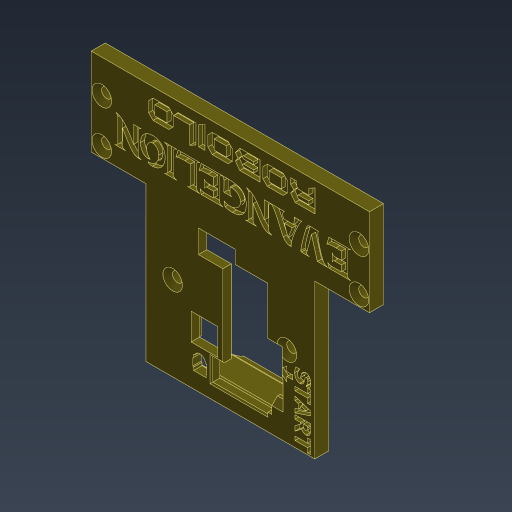
# Autodesk Inventor part: ceil
Saved by Autodesk Inventor 2023 (Build 270158000, 158)
## iProperties
Created: 2025-04-29
Part Number: ceil
Material: Generic
Document SubType Name: Modeling
Designer: szymo
Density: 1 g/cm^3
Appearance: Default(3)
Mass: 14.6413 g
Surface Area: 135.463 cm^2
Volume: 14.6413 cm^3
Author: szymo
Autodesk Inventor part; units mm, degrees
ref_plane "YZ Plane" through (0, 0, 0) normal (1, 0, 0) x (0, 1, 0)
ref_plane "XZ Plane" through (0, 0, 0) normal (0, 1, 0) x (-1, 0, 0)
ref_plane "XY Plane" through (0, 0, 0) normal (0, 0, 1) x (1, 0, 0)
ref_plane "Work Plane1" through (0, 0, 0) normal (0, 0, 1) x (1, 0, 0)
sketch "Sketch1" plane through (0, 0, 0) normal (0, 0, 1) x (1, 0, 0)
  spline S0 degree 2 poles (-9.1441, -18.5243) (-10.521, -19.0902) (-11.8979, -18.5243) knots 0 0 0 1 1 1 weights 1 1.096933 1
  line L0 (-16.1375, -18.5243) -> (-11.8979, -18.5243)
  line L1 (-16.1375, -20.5243) -> (-16.1375, -18.5243)
  line L2 (16.1375, -20.5243) -> (-16.1375, -20.5243)
  line L3 (16.1375, 6.7419) -> (16.1375, -20.5243)
  line L4 (16.1375, 6.7419) -> (16.1375, 10.5894)
  line L5 (8.6375, -18.5243) -> (8.6375, 6.7419)
  line L6 (-9.1441, -18.5243) -> (8.6375, -18.5243)
  circle A0 centre (12.3875, -16.7743) radius 2.75
  circle A1 centre (12.3875, -1.2581) radius 2.75
  line L7 (-53.5375, -20.5243) -> (-53.5375, -18.5243)
  line L8 (-53.5375, -18.5243) -> (-54.5271, -18.5243)
  line L9 (-54.5271, -18.5243) -> (-57.2809, -18.5243)
  line L10 (-57.2809, -18.5243) -> (-75.3625, -18.5243)
  line L11 (-75.3625, -18.5243) -> (-75.3625, 6.7419)
  line L12 (-82.8625, 6.7419) -> (-75.3625, 6.7419)
  line L13 (-82.8625, 6.7419) -> (-82.8625, -20.5243)
  line L14 (-82.8625, -20.5243) -> (-53.5375, -20.5243)
  circle A2 centre (-79.1125, -16.7743) radius 2.75
  circle A3 centre (-79.1125, -1.2581) radius 2.75
  arc A4 (-51.8547, -63.7607) -> (-50.5875, -61.8998) centre (-52.5875, -61.8998) ccw
  line L15 (-50.5875, -61.8998) -> (-50.5875, -36.1001)
  line L16 (-50.5875, -36.1001) -> (-56.7375, -36.1001)
  line L17 (-56.7375, -36.1001) -> (-56.7375, -20.5243)
  line L18 (-56.7375, -20.5243) -> (-61.3875, -20.5243)
  line L19 (-61.3875, -75.3243) -> (-61.3875, -20.5243)
  line L20 (-47.5875, -75.3243) -> (-61.3875, -75.3243)
  line L21 (-47.5875, -70.3243) -> (-47.5875, -75.3243)
  line L22 (-47.5875, -70.3243) -> (-50.6091, -70.3243)
  arc A5 (-51.8547, -63.7607) -> (-50.6091, -70.3243) centre (-50.6091, -66.9243) ccw
  circle A6 centre (-53.8875, -45.365) radius 2.75
  circle A7 centre (-13.2119, -46.6658) radius 2.75
  arc A8 (-14.1375, -70.3243) -> (-16.1375, -72.3243) centre (-14.1375, -72.3243) ccw
  line L23 (-16.1375, -72.3243) -> (-16.1375, -75.3243)
  line L24 (-16.1375, -75.3243) -> (-5.3375, -75.3243)
  line L25 (-5.3375, -20.5243) -> (-5.3375, -75.3243)
  line L26 (-16.1375, -20.5243) -> (-5.3375, -20.5243)
  line L27 (-16.1375, -58.1001) -> (-16.1375, -20.5243)
  line L28 (-16.1375, -58.1001) -> (-9.9875, -58.1001)
  line L29 (-9.9875, -58.1001) -> (-9.9875, -63.9243)
  arc A9 (-9.9875, -63.9243) -> (-10.3793, -65.8628) centre (-8.4794, -65.238) ccw
  arc A10 (-10.2091, -66.9243) -> (-10.3793, -65.8628) centre (-13.6102, -66.9254) ccw
  arc A11 (-13.6102, -70.3243) -> (-10.2091, -66.9243) centre (-13.6102, -66.9232) ccw
  line L30 (-13.6102, -70.3243) -> (-14.1375, -70.3243)
  line L31 (-5.3375, -75.3243) -> (-61.3875, -75.3243)
  line L32 (16.1375, 10.5894) -> (-82.3497, 10.5894)
  line L33 (-5.3375, -20.5243) -> (-5.3375, -75.3243)
  line L34 (-5.3375, -75.3243) -> (-3.3375, -75.3243)
  line L35 (-3.3375, -20.5243) -> (-3.3375, -75.3243)
  line L36 (-5.3375, -20.5243) -> (-3.3375, -20.5243)
  line L37 (-61.3875, -75.3243) -> (-61.3875, -20.5243)
  line L38 (-61.3875, -20.5243) -> (-63.3875, -20.5243)
  line L39 (-63.3875, -75.3243) -> (-63.3875, -73.1158)
  line L40 (-61.3875, -75.3243) -> (-63.3875, -75.3243)
  spline S1 degree 2 poles (-63.3875, -70.8783) (-63.0299, -71.9971) (-63.3875, -73.1158) knots 0 0 0 1 1 1 weights 1 1.055366 1
  line L41 (-63.3875, -70.8783) -> (-63.3875, -20.5243)
  line L42 (-63.3875, -73.1158) -> (-63.3875, -70.8783)
  line L43 (-22.0095, -69.5462) -> (-22.0095, -31.5462)
  line L44 (-34.0095, -69.5462) -> (-22.0095, -69.5462)
  line L45 (-34.0095, -31.5462) -> (-34.0095, -69.5462)
  line L46 (-22.0095, -31.5462) -> (-34.0095, -31.5462)
  line L47 (-41.7145, -65.6143) -> (-41.7145, -68.3743)
  line L48 (-41.7145, -68.3743) -> (-41.9645, -68.6243)
  line L49 (-41.9645, -68.6243) -> (-41.9645, -69.6243)
  line L50 (-41.9645, -69.6243) -> (-46.4645, -69.6243)
  line L51 (-46.4645, -69.6243) -> (-46.4645, -68.6243)
  line L52 (-46.4645, -68.6243) -> (-46.4645, -68.6243)
  line L53 (-46.7145, -68.3743) -> (-46.7145, -65.8743)
  line L54 (-46.7145, -65.8743) -> (-46.4645, -65.6243)
  line L55 (-46.4645, -65.6243) -> (-46.4645, -64.6243)
  line L56 (-46.4645, -68.6243) -> (-46.4645, -68.6243)
  line L57 (-46.4645, -68.6243) -> (-46.7145, -68.3743)
  line L58 (-42.7044, -64.6243) -> (-41.7145, -65.6143)
  line L59 (-46.4645, -64.6243) -> (-42.7044, -64.6243)
  line L60 (-36.1845, -69.2743) -> (-36.1845, -63.2743)
  line L61 (-36.1845, -69.2743) -> (-37.8845, -69.2743)
  line L62 (-39.0845, -68.4743) -> (-39.0845, -64.0743)
  line L63 (-36.1845, -63.2743) -> (-37.8845, -63.2743)
  line L64 (-37.8845, -63.2743) -> (-37.8845, -63.7743)
  line L65 (-38.7345, -63.7743) -> (-37.8845, -63.7743)
  line L66 (-38.7345, -63.7743) -> (-38.9845, -64.0243)
  line L67 (-37.8845, -69.2743) -> (-37.8845, -68.7743)
  line L68 (-38.9845, -68.5243) -> (-38.7345, -68.7743)
  line L69 (-38.7345, -68.7743) -> (-37.8845, -68.7743)
  line L70 (-38.9845, -68.5243) -> (-38.7345, -68.7743)
  line L71 (-38.9845, -68.4743) -> (-39.0845, -68.4743)
  line L72 (-38.9845, -68.4743) -> (-38.9845, -68.5243)
  line L73 (-38.9845, -64.0743) -> (-39.0845, -64.0743)
  line L74 (-38.9845, -64.0243) -> (-38.9845, -64.0743)
  line L75 (-38.8144, -60.2785) -> (-38.8144, -52.7785)
  line L76 (-46.3195, -60.2785) -> (-38.8144, -60.2785)
  line L77 (-46.3195, -52.7785) -> (-46.3195, -60.2785)
  line L78 (-38.8144, -52.7785) -> (-46.3195, -52.7785)
  line L79 (-32.6145, -25.8443) -> (-43.7145, -25.8443)
  line L80 (-43.7145, -25.8443) -> (-43.7145, -28.0943)
  line L81 (-43.7145, -28.0943) -> (-43.7145, -29.7943)
  line L82 (-43.7145, -25.8443) -> (-43.7145, -32.0443)
  line L83 (-43.7145, -32.0443) -> (-42.7145, -32.0443)
  line L84 (-42.7145, -32.0443) -> (-32.6145, -32.0443)
  line L85 (-42.7145, -32.0443) -> (-32.6145, -32.0443)
  line L86 (-32.6145, -25.8443) -> (-32.6145, -32.0443)
  line L87 (-17.8595, -56.3243) -> (-17.8595, -49.5243)
  line L88 (-20.8595, -56.3243) -> (-17.8595, -56.3243)
  line L89 (-20.8595, -49.5243) -> (-20.8595, -56.3243)
  line L90 (-17.8595, -49.5243) -> (-20.8595, -49.5243)
  line L91 (-17.6095, -63.5243) -> (-17.6095, -57.5243)
  line L92 (-17.6095, -63.5243) -> (-19.3095, -63.5243)
  line L93 (-19.3095, -63.5243) -> (-19.3095, -63.0243)
  line L94 (-20.1595, -63.0243) -> (-19.3095, -63.0243)
  line L95 (-20.4095, -62.7743) -> (-20.1595, -63.0243)
  line L96 (-20.4095, -62.7243) -> (-20.4095, -62.7743)
  line L97 (-20.4095, -62.7243) -> (-20.5095, -62.7243)
  line L98 (-20.4095, -62.7243) -> (-20.5095, -62.7243)
  line L99 (-20.5095, -62.7243) -> (-20.5095, -58.3243)
  line L100 (-17.6095, -57.5243) -> (-19.3095, -57.5243)
  line L101 (-19.3095, -57.5243) -> (-19.3095, -58.0243)
  line L102 (-20.1595, -58.0243) -> (-19.3095, -58.0243)
  line L103 (-20.1595, -58.0243) -> (-20.4095, -58.2743)
  line L104 (-20.4095, -58.2743) -> (-20.4095, -58.3243)
  line L105 (-20.4095, -58.3243) -> (-20.5095, -58.3243)
  line L106 (-19.6095, -66.9243) -> (-19.6095, -66.6743)
  line L107 (-19.6095, -66.3743) -> (-19.6095, -66.1243)
  line L108 (-19.9095, -66.1243) -> (-20.9095, -66.1243)
  line L109 (-21.2095, -66.3743) -> (-21.2095, -66.1243)
  line L110 (-21.2095, -66.9243) -> (-21.2095, -66.6743)
  line L111 (-19.9095, -66.9243) -> (-20.9095, -66.9243)
  line L112 (-19.9095, -67.4743) -> (-20.9095, -67.4743)
  line L113 (-19.9095, -68.2743) -> (-20.9095, -68.2743)
  line L114 (-19.6095, -68.2743) -> (-19.6095, -68.0243)
  line L115 (-19.6095, -67.7243) -> (-19.6095, -67.4743)
  line L116 (-21.2095, -67.7243) -> (-21.2095, -67.4743)
  line L117 (-21.2095, -68.2743) -> (-21.2095, -68.0243)
  line L118 (-19.6095, -65.6243) -> (-19.6095, -65.3743)
  line L119 (-19.6095, -65.0743) -> (-19.6095, -64.8243)
  line L120 (-19.9095, -64.8243) -> (-20.9095, -64.8243)
  line L121 (-19.9095, -65.6243) -> (-20.9095, -65.6243)
  line L122 (-21.2095, -65.6243) -> (-21.2095, -65.3743)
  line L123 (-21.2095, -65.0743) -> (-21.2095, -64.8243)
  line L124 (-20.0095, -70.2743) -> (-20.0095, -29.5462)
  line L125 (-20.0095, -29.5462) -> (-36.0095, -29.5462)
  line L126 (-36.0095, -29.5462) -> (-36.0095, -70.2743)
  line L127 (-31.6145, -24.8443) -> (-44.7145, -24.8443)
  line L128 (-44.7145, -24.8443) -> (-44.7145, -33.0443)
  line L129 (-44.7145, -33.0443) -> (-31.6145, -33.0443)
  line L130 (-31.6145, -33.0443) -> (-31.6145, -24.8443)
  line L131 (-21.8595, -48.5243) -> (-21.8595, -57.3243)
  line L132 (-21.8595, -57.3243) -> (-16.8595, -57.3243)
  line L133 (-16.8595, -57.3243) -> (-16.8595, -48.5243)
  line L134 (-16.8595, -48.5243) -> (-21.8595, -48.5243)
  line L135 (-16.6095, -64.5243) -> (-21.5095, -64.5243)
  line L136 (-21.5095, -64.5243) -> (-21.5095, -56.5243)
  line L137 (-21.5095, -56.5243) -> (-16.6095, -56.5243)
  line L138 (-16.6095, -56.5243) -> (-16.6095, -64.5243)
  line L139 (-40.0845, -70.2743) -> (-35.1845, -70.2743)
  line L140 (-35.1845, -70.2743) -> (-35.1845, -62.2743)
  line L141 (-35.1845, -62.2743) -> (-40.0845, -62.2743)
  line L142 (-40.0845, -62.2743) -> (-40.0845, -70.2743)
  line L143 (-37.8144, -61.2785) -> (-37.8144, -51.7785)
  line L144 (-37.8144, -51.7785) -> (-47.3195, -51.7785)
  line L145 (-47.3195, -51.7785) -> (-47.3195, -61.2785)
  line L146 (-47.3195, -61.2785) -> (-37.8144, -61.2785)
  circle A12 centre (-44.2145, -65.3243) radius 0.4
  circle A13 centre (-44.2145, -65.3243) radius 2
  line L147 (-18.6095, -69.2743) -> (-22.2095, -69.2743)
  line L148 (-22.2095, -69.2743) -> (-22.2095, -64.5243)
  line L149 (-22.2095, -64.5243) -> (-18.6095, -64.5243)
  line L150 (-18.6095, -64.5243) -> (-18.6095, -69.2743)
  line L151 (-82.8625, 10.5894) -> (-75.3625, 10.5894)
  line L152 (-82.8625, 6.7419) -> (-82.8625, 10.5894)
  line L153 (-20.0095, -70.2743) -> (-36.0095, -70.2743)
  line L154 (-36.0095, -70.2743) -> (-41.4052, -70.2743) construction
  point P0 (0, 0)
  point P1 (-37.6345, -70.2743)
  point P2 (-36.0095, -70.2743)
  point P3 (-36.0095, -62.2743)
  point P4 (-36.0095, -33.0443)
  point P5 (-31.6145, -29.5462)
  point P6 (-20.0095, -48.5243)
  point P7 (-16.6095, -58.3243)
  point P8 (-20.0095, -69.2743)
  point P9 (-42.8879, -64.6243)
  point P10 (-46.088, -64.6243)
  point P11 (-20.0095, -64.5243)
  point P12 (-16.8595, -56.5243)
  point P13 (-20.0095, -56.5243)
  point P14 (-20.0095, -57.3243)
  point P15 (-21.5095, -57.3243)
  point P16 (-42.2269, -65.1019)
  dimension "d97" = 1
  dimension "d98" = 1
  dimension "d99" = 1
  dimension "d100" = 1
  dimension "d101" = 1
  dimension "d102" = 1
  dimension "d103" = 4
  dimension "d104" = 1
  dimension "d105" = 1
  dimension "d106" = 1
  dimension "d107" = 1
  dimension "d108" = 1
  dimension "d109" = 1
  dimension "d110" = 1
  dimension "d111" = 1
  dimension "d112" = 1
  dimension "d113" = 1
  dimension "d114" = 1
  dimension "d153" = 2
  dimension "d154" = 0.7281
  dimension "d155" = 0
  constraints: 234 end point, 15 vertical, 12 horizontal, 11 parallel, 6 perpendicular, 3 collinear, 2 centre point, 1 coincident, 1 midpoint, 1 point on line, 165 other
  measures "d97" distance between parallel lines of L127 L79
  measures "d98" distance between parallel lines of L128 L80
  measures "d99" distance between parallel lines of L129 L84
  measures "d100" distance between parallel lines of L130 L86
  measures "d101" distance between parallel lines of L90 L134
  measures "d102" distance between parallel lines of L76 L146
  measures "d103" diameter of A13
  measures "d104" distance between parallel lines of L138 L91
  measures "d105" distance between parallel lines of L135 L92
  measures "d106" distance between parallel lines of L136 L99
  measures "d107" distance between parallel lines of L100 L137
  measures "d108" distance from line of L61 point (-37.635, -70.274)
  measures "d109" distance between parallel lines of L142 L62
  measures "d110" distance between parallel lines of L63 L141
  measures "d111" distance between parallel lines of L140 L60
  measures "d112" distance between parallel lines of L150 L114
  measures "d113" distance between parallel lines of L147 L113
  measures "d114" distance from line of L148 L117.end
  measures "d153" distance between parallel lines of L45 L126
  measures "d154" distance between parallel lines of L153 L44
  measures "d155" distance between parallel lines of L154 L139
extrude "Extrusion1" add sketch "Sketch1" along normal blind 5 contours L2 L27 L28 L29 A9 A10 A11 L30 A8 L23 L31 L21 L22 A5 A4 L15 L16 L17 L14 L7 L8 L9 L10 L11 L12 L152 L151 L32 L4 L3 | L35 L34 L25 L2 | L25 L24 L23 A8 L30 A11 A10 A9 L29 L28 L27 L2 | L20 L19 L14 L17 L16 L15 A4 A5 L22 L21 | L40 L39 S1 L41 L14 L19 | L12 L11 L10 L9 L8 L7 L14 L13 | L42 S1 | A0 | A1 | A2 | A3 | A6 | A7
sketch "Sketch6" plane through (0, 0, 0) normal (0, 0, -1) x (-1, 0, 0)
  circle A0 centre (50.6091, -66.9243) radius 2
  arc A1 (16.1375, -65.8429) -> (16.1375, -68.0058) centre (13.6091, -66.9243) ccw
  circle A2 centre (50.6091, -66.9243) radius 4
  circle A3 centre (13.6091, -66.9243) radius 3.5
  point P0 (0, 0)
  dimension "d83" = 8
  dimension "d84" = 7
  constraints: 4 centre point, 2 coincident, 2 point on circle, 6 other
  measures "d83" diameter of A2
  measures "d84" diameter of A3
extrude "Extrusion5" cut sketch "Sketch6" against normal blind 2 contours A0 | A2 | A3
ref_plane "Work Plane2" through (-16.6375, -70.0451, -5.2063) normal (-1, 0, 0) x (0, -0.9586871, -0.2844628)
sketch "Sketch7" plane through (-16.6375, -70.0451, -5.2063) normal (-1, 0, 0) x (0, -0.9586871, -0.2844628)
  line L0 (3.5801, 6.493) -> (7.0645, -5.2498)
  arc A0 (6.3902, -6.493) -> (-6.4635, -1.1345) centre (-4.8206, -15.2895) ccw
  line L1 (-0.6539, 3.1854) -> (-1.2133, 5.0707)
  line L2 (7.3489, -6.2085) -> (6.3902, -6.493)
  line L3 (1.4628, 5.8648) -> (3.5801, 6.493)
  line L4 (-0.6822, 5.2283) -> (1.4628, 5.8648)
  line L5 (-0.6822, 5.2283) -> (-1.2133, 5.0707)
  line L6 (-0.1588, 5.3836) -> (2.3155, -2.9551)
  line L7 (7.0645, -5.2498) -> (7.3489, -6.2085)
  line L8 (-0.1588, 5.3836) -> (-1.2133, 5.0707)
  point P0 (-68.6323, -14.934)
  dimension "d88" = 1
  dimension "d89" = 1.1
  dimension "d150" = 3.9
  constraints: 18 end point, 4 point on circle, 2 perpendicular, 2 point on line, 1 centre point, 1 collinear, 14 other
  measures "d88" distance of L2.start L2.end
  measures "d89" distance between parallel lines of L1 L6
  measures "d150" distance between parallel lines of L6 L0
extrude "Extrusion6" add sketch "Sketch7" along normal blind 30.45
chamfer "Chamfer8" distance 2 angle 45 4 edges at (-18.4345, -48.5243, 5) (-16.8595, -52.5243, 5) (-16.6095, -60.5243, 5) (-17.6095, -64.5243, 5)
chamfer "Chamfer9" distance 0.5 angle 45 3 edges at (-30.047, -70.2743, 5) (-40.0845, -66.2743, 5) (-38.047, -62.2743, 5)
sketch "Sketch5" plane through (0, 0, 5) normal (0, 0, 1) x (1, 0, 0)
  spline S0 degree 2 poles (-9.1441, -18.5243) (-10.521, -19.0902) (-11.8979, -18.5243) knots 0 0 0 1 1 1 weights 1 1.096933 1
  line L0 (-16.1375, -18.5243) -> (-11.8979, -18.5243)
  line L1 (-16.1375, -20.5243) -> (-16.1375, -18.5243)
  line L2 (16.1375, -20.5243) -> (-16.1375, -20.5243)
  line L3 (16.1375, 6.7419) -> (16.1375, -20.5243)
  line L4 (16.1375, 6.7419) -> (8.6375, 6.7419)
  line L5 (8.6375, -18.5243) -> (8.6375, 6.7419)
  line L6 (-9.1441, -18.5243) -> (8.6375, -18.5243)
  circle A0 centre (12.3875, -16.7743) radius 2.75
  circle A1 centre (12.3875, -1.2581) radius 2.75
  line L7 (-53.5375, -20.5243) -> (-53.5375, -18.5243)
  line L8 (-53.5375, -18.5243) -> (-54.5271, -18.5243)
  line L9 (-54.5271, -18.5243) -> (-57.2809, -18.5243)
  line L10 (-57.2809, -18.5243) -> (-75.3625, -18.5243)
  line L11 (-75.3625, -18.5243) -> (-75.3625, 6.7419)
  line L12 (-82.8625, 6.7419) -> (-75.3625, 6.7419)
  line L13 (-82.8625, 6.7419) -> (-82.8625, -20.5243)
  line L14 (-82.8625, -20.5243) -> (-53.5375, -20.5243)
  circle A2 centre (-79.1125, -16.7743) radius 2.75
  circle A3 centre (-79.1125, -1.2581) radius 2.75
  arc A4 (-51.8547, -63.7607) -> (-50.5875, -61.8998) centre (-52.5875, -61.8998) ccw
  line L15 (-50.5875, -61.8998) -> (-50.5875, -36.1001)
  line L16 (-50.5875, -36.1001) -> (-56.7375, -36.1001)
  line L17 (-56.7375, -36.1001) -> (-56.7375, -20.5243)
  line L18 (-56.7375, -20.5243) -> (-61.3875, -20.5243)
  line L19 (-61.3875, -75.3243) -> (-61.3875, -20.5243)
  line L20 (-47.5875, -75.3243) -> (-61.3875, -75.3243)
  line L21 (-47.5875, -70.3243) -> (-47.5875, -75.3243)
  line L22 (-47.5875, -70.3243) -> (-50.6091, -70.3243)
  arc A5 (-51.8547, -63.7607) -> (-50.6091, -70.3243) centre (-50.6091, -66.9243) ccw
  circle A6 centre (-53.8875, -45.365) radius 2.75
  circle A7 centre (-13.2119, -46.6658) radius 2.75
  arc A8 (-14.1375, -70.3243) -> (-16.1375, -72.3243) centre (-14.1375, -72.3243) ccw
  line L23 (-16.1375, -72.3243) -> (-16.1375, -75.3243)
  line L24 (-16.1375, -75.3243) -> (-5.3375, -75.3243)
  line L25 (-5.3375, -20.5243) -> (-5.3375, -75.3243)
  line L26 (-16.1375, -20.5243) -> (-5.3375, -20.5243)
  line L27 (-16.1375, -58.1001) -> (-16.1375, -20.5243)
  line L28 (-16.1375, -58.1001) -> (-9.9875, -58.1001)
  line L29 (-9.9875, -58.1001) -> (-9.9875, -63.9243)
  arc A9 (-9.9875, -63.9243) -> (-10.3793, -65.8628) centre (-8.4794, -65.238) ccw
  arc A10 (-10.2091, -66.9243) -> (-10.3793, -65.8628) centre (-13.6102, -66.9254) ccw
  arc A11 (-13.6102, -70.3243) -> (-10.2091, -66.9243) centre (-13.6102, -66.9232) ccw
  line L30 (-13.6102, -70.3243) -> (-14.1375, -70.3243)
  point P0 (0, 0)
  point P1 (12.3875, -1.2581)
  point P2 (12.3875, -16.7743)
  dimension "d108" = 1
  constraints: 8 coincident
hole "Hole1" at (-53.8875, -45.365, 5) at (-13.2119, -46.6658, 5) at (12.3875, -1.2581, 5) at (12.3875, -16.7743, 5) at (-79.1125, -16.7743, 5) at (-79.1125, -1.2581, 5) direction (0, 0, -1) diameter 3.6 depth 8.8 countersink diameter 7 countersink angle 90 clearance for "Countersunk Flat Head Screw ISO 2009/7046" size "M3" standard "ISO"
fillet "Fillet1" radius 0.6 8 edges at (-47.0875, -71.4243, -4.349) (-47.0875, -73.0917, -10.8349) (-47.0875, -74.8243, -13.2489) (-16.6375, -73.0917, -10.8349) (-16.6375, -71.4243, -4.349) (-16.6375, -74.8243, -13.2489) (-31.8625, -74.3243, -13.2489) (-31.8625, -71.4243, -8.698)
sketch "Sketch8" plane through (0, 0, 0) normal (0, 0, -1) x (-1, 0, 0)
  line L0 (50.6091, -69.9243) -> (13.6091, -69.9243)
  arc A0 (50.6091, -69.9243) -> (50.6091, -63.9243) centre (50.6091, -66.9243) ccw
  line L1 (49.1091, -63.9243) -> (50.6091, -63.9243)
  arc A1 (47.1091, -61.9243) -> (49.1091, -63.9243) centre (49.1098, -61.9236) ccw
  line L2 (47.1091, -17.9243) -> (47.1091, -61.9243)
  line L3 (17.1091, -17.9243) -> (47.1091, -17.9243)
  line L4 (17.1091, -61.9243) -> (17.1091, -17.9243)
  arc A2 (15.1091, -63.9243) -> (17.1091, -61.9243) centre (15.1083, -61.9236) ccw
  line L5 (13.6091, -63.9243) -> (15.1091, -63.9243)
  arc A3 (13.6091, -63.9243) -> (10.6091, -66.9243) centre (13.6102, -66.9254) ccw
  arc A4 (10.6091, -66.9243) -> (13.6091, -69.9243) centre (13.6102, -66.9232) ccw
  line L6 (48.6091, -62.4243) -> (50.6091, -62.4243)
  arc A5 (50.6091, -71.4243) -> (50.6091, -62.4243) centre (50.6091, -66.9243) ccw
  line L7 (50.6091, -71.4243) -> (13.6102, -71.4243)
  arc A6 (9.1091, -66.9243) -> (13.6102, -71.4243) centre (13.6102, -66.9232) ccw
  arc A7 (13.6102, -62.4243) -> (9.1091, -66.9243) centre (13.6102, -66.9254) ccw
  line L8 (13.6102, -62.4243) -> (15.6091, -62.4243)
  line L9 (15.6091, -62.4243) -> (15.6091, -16.4243)
  line L10 (15.6091, -16.4243) -> (48.6091, -16.4243)
  line L11 (48.6091, -16.4243) -> (48.6091, -62.4243)
  arc A8 (46.7145, -67.8366) -> (46.7145, -66.012) centre (50.6091, -66.9243) ccw projected
  circle A9 centre (13.6091, -66.9243) radius 3.5 projected
  line L12 (48.6091, -62.4243) -> (48.6091, -63.4602)
  arc A10 (46.7145, -67.8366) -> (46.7145, -66.012) centre (50.6091, -66.9243) ccw projected
  line L13 (15.6091, -62.4243) -> (15.6091, -64.052)
  line L14 (50.6091, -70.9243) -> (13.5618, -70.424)
  circle A11 centre (13.6091, -66.9243) radius 3.5 projected
  point P0 (0, 0)
  point P1 (13.5618, -70.424)
  point P2 (48.5019, -70.3243)
  point P3 (50.8752, -62.9332)
  point P4 (50.5011, -70.9229)
  dimension "d93" = 1.5
  constraints: 30 end point, 19 point on circle, 8 centre point, 4 horizontal, 3 vertical, 1 perpendicular, 1 tangent, 32 other
  measures "d93" distance between parallel lines of L2 L11
extrude "Extrusion7" cut sketch "Sketch8" against normal blind 2
sketch "Sketch4" plane through (0, 0, 5) normal (0, 0, 1) x (1, 0, 0)
  line L0 (11.6625, -12.3333) -> (-78.3875, -12.3333) construction
  line L1 (-78.3875, -12.3333) -> (-78.3875, -5.6552) construction
  line L2 (-78.3875, -5.6552) -> (11.6625, -5.6552) construction
  line L3 (11.6625, -5.6552) -> (11.6625, -12.3333) construction
  line L4 (-82.8625, -20.5243) -> (-63.3875, -20.5243) projected
  line L5 (-3.3375, -75.3243) -> (-3.3375, -20.5243) projected
  line L6 (-3.3375, -20.5243) -> (16.1375, -20.5243) projected
  line L7 (11.6625, 1.1251) -> (-78.3875, 1.1251) construction
  line L8 (-78.3875, 1.1251) -> (-78.3875, 6.1749) construction
  line L9 (-78.3875, 6.1749) -> (11.6625, 6.1749) construction
  line L10 (11.6625, 6.1749) -> (11.6625, 1.1251) construction
  line L11 (-63.3875, -20.5243) -> (-63.3875, -75.3243) projected
  line L12 (-63.3875, -75.3243) -> (-3.3375, -75.3243) projected
  line L13 (16.1375, -20.5243) -> (16.1375, 10.5894) projected
  line L14 (16.1375, 10.5894) -> (-82.8625, 10.5894) projected
  line L15 (-82.8625, 10.5894) -> (-82.8625, -20.5243) projected
  line L16 (-11.9108, 7.0782) -> (-9.681, 7.0782)
  line L17 (-9.681, 7.0782) -> (-9.681, 5.3968)
  line L18 (-9.681, 5.3968) -> (-9.1327, 4.8641)
  line L19 (-9.1327, 4.8641) -> (-5.4722, 4.8641)
  line L20 (-5.4722, 4.8641) -> (-5.4722, 7.0312)
  line L21 (-5.4722, 7.0312) -> (-3.2424, 8.2271)
  line L22 (-3.2424, 8.2271) -> (-3.2424, 0.2271)
  line L23 (-3.2424, 0.2271) -> (-10.3442, 0.2271)
  line L24 (-10.3442, 0.2271) -> (-11.9108, 2.3785)
  line L25 (-11.9108, 2.3785) -> (-10.762, 3.9085)
  line L26 (-10.762, 3.9085) -> (-11.9108, 5.0208)
  line L27 (-11.9108, 5.0208) -> (-11.9108, 7.0782)
  line L28 (-9.6236, 2.509) -> (-9.1484, 1.9242)
  line L29 (-9.1484, 1.9242) -> (-5.4722, 1.9242)
  line L30 (-5.4722, 1.9242) -> (-5.4722, 3.1304)
  line L31 (-5.4722, 3.1304) -> (-9.1432, 3.1304)
  line L32 (-9.1432, 3.1304) -> (-9.6236, 2.509)
  line L33 (-21.7803, 5.5064) -> (-20.2085, 7.0782)
  line L34 (-20.2085, 7.0782) -> (-14.5844, 7.0782)
  line L35 (-14.5844, 7.0782) -> (-13.0126, 5.5064)
  line L36 (-13.0126, 5.5064) -> (-13.0126, 1.7989)
  line L37 (-13.0126, 1.7989) -> (-14.5844, 0.2271)
  line L38 (-14.5844, 0.2271) -> (-20.2085, 0.2271)
  line L39 (-20.2085, 0.2271) -> (-21.7803, 1.7989)
  line L40 (-21.7803, 1.7989) -> (-21.7803, 5.5064)
  line L41 (-19.5505, 5.3811) -> (-19.5505, 1.9242)
  line L42 (-19.5505, 1.9242) -> (-15.2424, 1.9242)
  line L43 (-15.2424, 1.9242) -> (-15.2424, 5.3811)
  line L44 (-15.2424, 5.3811) -> (-19.5505, 5.3811)
  line L45 (-31.5766, 4.9425) -> (-30.01, 7.0887)
  line L46 (-30.01, 7.0887) -> (-22.8194, 7.0887)
  line L47 (-22.8194, 7.0887) -> (-22.8194, 0.2271)
  line L48 (-22.8194, 0.2271) -> (-30.01, 0.2271)
  line L49 (-30.01, 0.2271) -> (-31.5766, 2.3733)
  line L50 (-31.5766, 2.3733) -> (-30.6314, 3.6579)
  line L51 (-30.6314, 3.6579) -> (-31.5766, 4.9425)
  line L52 (-29.1536, 2.3785) -> (-28.7306, 1.9346)
  line L53 (-28.7306, 1.9346) -> (-25.0492, 1.9346)
  line L54 (-25.0492, 1.9346) -> (-25.0492, 2.8746)
  line L55 (-25.0492, 2.8746) -> (-28.7254, 2.8746)
  line L56 (-28.7254, 2.8746) -> (-29.1536, 2.3785)
  line L57 (-29.1536, 4.9372) -> (-28.7254, 4.4464)
  line L58 (-28.7254, 4.4464) -> (-25.0492, 4.4464)
  line L59 (-25.0492, 4.4464) -> (-25.0492, 5.3811)
  line L60 (-25.0492, 5.3811) -> (-28.7306, 5.3811)
  line L61 (-28.7306, 5.3811) -> (-29.1536, 4.9372)
  line L62 (-41.3573, 5.5064) -> (-39.7855, 7.0782)
  line L63 (-39.7855, 7.0782) -> (-34.1615, 7.0782)
  line L64 (-34.1615, 7.0782) -> (-32.5897, 5.5064)
  line L65 (-32.5897, 5.5064) -> (-32.5897, 1.7989)
  line L66 (-32.5897, 1.7989) -> (-34.1615, 0.2271)
  line L67 (-34.1615, 0.2271) -> (-39.7855, 0.2271)
  line L68 (-39.7855, 0.2271) -> (-41.3573, 1.7989)
  line L69 (-41.3573, 1.7989) -> (-41.3573, 5.5064)
  line L70 (-39.1275, 5.3811) -> (-39.1275, 1.9242)
  line L71 (-39.1275, 1.9242) -> (-34.8194, 1.9242)
  line L72 (-34.8194, 1.9242) -> (-34.8194, 5.3811)
  line L73 (-34.8194, 5.3811) -> (-39.1275, 5.3811)
  line L74 (-44.6262, 7.0417) -> (-42.3964, 8.2271)
  line L75 (-42.3964, 8.2271) -> (-42.3964, 0.2271)
  line L76 (-42.3964, 0.2271) -> (-44.6262, 0.2271)
  line L77 (-44.6262, 0.2271) -> (-44.6262, 7.0417)
  line L78 (-53.5244, 5.3811) -> (-51.9735, 7.0887)
  line L79 (-51.9735, 7.0887) -> (-45.6027, 7.0887)
  line L80 (-45.6027, 7.0887) -> (-45.6027, 0.2793)
  line L81 (-45.6027, 0.2793) -> (-47.8325, -0.9322)
  line L82 (-47.8325, -0.9322) -> (-47.8325, 5.3811)
  line L83 (-47.8325, 5.3811) -> (-53.5244, 5.3811)
  line L84 (-62.4539, 5.5064) -> (-60.8821, 7.0782)
  line L85 (-60.8821, 7.0782) -> (-55.2581, 7.0782)
  line L86 (-55.2581, 7.0782) -> (-53.6863, 5.5064)
  line L87 (-53.6863, 5.5064) -> (-53.6863, 1.7989)
  line L88 (-53.6863, 1.7989) -> (-55.2581, 0.2271)
  line L89 (-55.2581, 0.2271) -> (-60.8821, 0.2271)
  line L90 (-60.8821, 0.2271) -> (-62.4539, 1.7989)
  line L91 (-62.4539, 1.7989) -> (-62.4539, 5.5064)
  line L92 (-60.2241, 5.3811) -> (-60.2241, 1.9242)
  line L93 (-60.2241, 1.9242) -> (-55.916, 1.9242)
  line L94 (-55.916, 1.9242) -> (-55.916, 5.3811)
  line L95 (-55.916, 5.3811) -> (-60.2241, 5.3811)
  line L96 (1.7228, -4.4618) -> (0.9378, -7.0352)
  spline S0 degree 2 poles (0.9378, -7.0352) (1.0744, -6.8236) (2.0983, -6.5983) (3.4976, -6.5232) (4.2143, -6.5232) knots 0 0 0 1 2 3 3 3
  spline S1 degree 2 poles (4.2143, -6.5232) (4.8628, -6.5232) (5.8866, -6.5506) (6.146, -6.5506) knots 0 0 0 1 2 2 2
  line L97 (6.146, -6.5506) -> (6.146, -9.4243)
  line L98 (6.146, -9.4243) -> (3.7023, -9.4243)
  spline S2 degree 2 poles (3.7023, -9.4243) (3.3679, -9.3355) (2.9242, -9.0011) (2.8832, -8.728) knots 0 0 0 1 2 2 2
  line L99 (2.8832, -8.728) -> (2.8832, -11.513)
  spline S3 degree 2 poles (2.8832, -11.513) (2.931, -11.24) (3.3337, -10.8987) (3.6546, -10.8168) knots 0 0 0 1 2 2 2
  line L100 (3.6546, -10.8168) -> (6.146, -10.8168)
  line L101 (6.146, -10.8168) -> (6.146, -12.8782)
  spline S4 degree 2 poles (6.146, -12.8782) (5.9344, -12.885) (5.2041, -12.9123) (4.2757, -12.9465) (3.7843, -12.9465) knots 0 0 0 1 2 3 3 3
  spline S5 degree 2 poles (3.7843, -12.9465) (3.2041, -12.9465) (2.1597, -12.8645) (1.4225, -12.6529) (1.2996, -12.4482) knots 0 0 0 1 2 3 3 3
  line L102 (1.2996, -12.4482) -> (1.7228, -14.0181)
  line L103 (1.7228, -14.0181) -> (9.4498, -14.0181)
  spline S6 degree 2 poles (9.4498, -14.0181) (9.1017, -13.9703) (8.5419, -13.6495) (8.3372, -13.3492) knots 0 0 0 1 2 2 2
  line L104 (8.3372, -13.3492) -> (8.3372, -5.1171)
  spline S7 degree 2 poles (8.3372, -5.1171) (8.5419, -4.8236) (9.1017, -4.5096) (9.4498, -4.4618) knots 0 0 0 1 2 2 2
  line L105 (9.4498, -4.4618) -> (1.7228, -4.4618)
  spline S8 degree 2 poles (-4.2567, -4.4482) (-4.4478, -4.4482) (-4.8164, -4.4686) (-4.9939, -4.4755) knots 0 0 0 1 2 2 2
  spline S9 degree 2 poles (-4.9939, -4.4755) (-5.499, -4.5232) (-6.0178, -4.8236) (-6.3045, -5.4789) (-6.482, -6.0659) knots 0 0 0 1 2 3 3 3
  spline S10 degree 2 poles (-6.482, -6.0659) (-6.6799, -6.728) (-7.1577, -8.3799) (-7.6287, -10.1546) (-8.0178, -11.8202) (-8.2499, -13.1717) (-8.2567, -13.5744) knots 0 0 0 1 2 3 4 5 5 5
  spline S11 degree 2 poles (-8.2567, -13.5744) (-8.2567, -13.7587) (-8.1816, -13.9772) (-8.1134, -13.9908) knots 0 0 0 1 2 2 2
  line L106 (-8.1134, -13.9908) -> (-5.2942, -13.9908)
  spline S12 degree 2 poles (-5.2942, -13.9908) (-5.5878, -13.9499) (-6.086, -13.711) (-6.284, -13.4925) knots 0 0 0 1 2 2 2
  spline S13 degree 2 poles (-6.284, -13.4925) (-5.9837, -12.2639) (-5.3898, -10.1069) (-4.8028, -7.9635) (-4.5093, -6.7622) knots 0 0 0 1 2 3 3 3
  line L107 (-4.5093, -6.7622) -> (-2.4069, -14.0181)
  line L108 (-2.4069, -14.0181) -> (1.2382, -14.0181)
  spline S14 degree 2 poles (1.2382, -14.0181) (1.1153, -13.9908) (0.5215, -13.7383) (-0.011, -13.4379) (-0.0587, -13.3355) knots 0 0 0 1 2 3 3 3
  spline S15 degree 2 poles (-0.0587, -13.3355) (-0.1475, -13.2673) (-0.6321, -12.1205) (-1.2533, -10.3458) (-1.8403, -8.2912) (-2.2294, -6.3185) (-2.2362, -5.5608) knots 0 0 0 1 2 3 4 5 5 5
  spline S16 degree 2 poles (-2.2362, -5.5608) (-2.2362, -5.2127) (-2.1338, -4.6802) (-2.0246, -4.5028) knots 0 0 0 1 2 2 2
  spline S17 degree 2 poles (-2.0246, -4.5028) (-2.6321, -4.5028) (-3.6219, -4.4686) (-4.011, -4.4482) knots 0 0 0 1 2 2 2
  line L109 (-4.011, -4.4482) -> (-4.2567, -4.4482)
  spline S18 degree 2 poles (-18.8779, -4.4618) (-18.5024, -4.6598) (-17.7174, -5.7383) (-16.9256, -7.2605) (-16.1543, -8.9806) (-15.4376, -10.6666) (-14.7959, -12.0659) (-14.5297, -12.5028) knots 0 0 0 1 2 3 4 5 6 6 6
  spline S19 degree 2 poles (-14.5297, -12.5028) (-14.1134, -13.1649) (-13.2874, -13.868) (-12.557, -14.1137) (-12.2703, -14.1069) knots 0 0 0 1 2 3 3 3
  spline S20 degree 2 poles (-12.2703, -14.1069) (-12.0178, -14.1) (-11.697, -14.0181) (-11.656, -14.0045) knots 0 0 0 1 2 2 2
  spline S21 degree 2 poles (-11.656, -14.0045) (-11.697, -13.9362) (-11.7243, -13.7246) (-11.7243, -13.6017) knots 0 0 0 1 2 2 2
  spline S22 degree 2 poles (-11.7243, -13.6017) (-11.7174, -13.0762) (-11.2738, -11.3628) (-10.5434, -9.3219) (-9.6765, -7.2741) (-8.8233, -5.5608) (-8.1407, -4.5096) (-7.9495, -4.4755) knots 0 0 0 1 2 3 4 5 6 6 6
  line L110 (-7.9495, -4.4755) -> (-10.7209, -4.4755)
  spline S23 degree 2 poles (-10.7209, -4.4755) (-10.6321, -4.4823) (-10.5639, -4.7144) (-10.5639, -4.9055) knots 0 0 0 1 2 2 2
  spline S24 degree 2 poles (-10.5639, -4.9055) (-10.5639, -5.2263) (-10.6867, -6.0181) (-10.8369, -6.7075) (-10.8915, -6.8645) knots 0 0 0 1 2 3 3 3
  line L111 (-10.8915, -6.8645) -> (-14.5024, -6.8645)
  spline S25 degree 2 poles (-14.5024, -6.8645) (-14.5775, -6.5574) (-14.7209, -5.9157) (-14.7277, -5.5949) knots 0 0 0 1 2 2 2
  spline S26 degree 2 poles (-14.7277, -5.5949) (-14.7345, -5.2536) (-14.4547, -4.6734) (-14.0997, -4.4755) knots 0 0 0 1 2 2 2
  line L112 (-14.0997, -4.4755) -> (-18.8779, -4.4618)
  line L113 (-14.168, -8.1273) -> (-11.3557, -8.1273)
  spline S27 degree 2 poles (-11.3557, -8.1273) (-11.6082, -8.8031) (-12.1475, -10.1751) (-12.6321, -11.3901) (-12.8233, -11.8338) knots 0 0 0 1 2 3 3 3
  spline S28 degree 2 poles (-12.8233, -11.8338) (-13.1645, -10.926) (-13.8608, -9.0625) (-14.168, -8.1273) knots 0 0 0 1 2 2 2
  spline S29 degree 2 poles (-27.5809, -3.8748) (-27.5673, -3.8816) (-27.226, -4.1683) (-26.8847, -4.6052) (-26.8779, -4.8441) knots 0 0 0 1 2 3 3 3
  line L114 (-26.8779, -4.8441) -> (-26.8779, -13.3355)
  spline S30 degree 2 poles (-26.8779, -13.3355) (-27.0826, -13.6427) (-27.656, -13.9703) (-27.9973, -14.0181) knots 0 0 0 1 2 2 2
  line L115 (-27.9973, -14.0181) -> (-24.1202, -14.0181)
  spline S31 degree 2 poles (-24.1202, -14.0181) (-24.4683, -13.9703) (-25.0349, -13.6427) (-25.2465, -13.3355) knots 0 0 0 1 2 2 2
  line L116 (-25.2465, -13.3355) -> (-25.2465, -7.6086)
  spline S32 degree 2 poles (-25.2465, -7.6086) (-24.912, -8.0727) (-24.0314, -9.6222) (-22.9734, -11.3901) (-21.7652, -12.9874) (-20.4547, -13.9977) (-19.7584, -14.0181) knots 0 0 0 1 2 3 4 5 5 5
  line L117 (-19.7584, -14.0181) -> (-18.5707, -14.0181)
  spline S33 degree 2 poles (-18.5707, -14.0181) (-18.9188, -13.9703) (-19.4785, -13.6564) (-19.6833, -13.3628) knots 0 0 0 1 2 2 2
  line L118 (-19.6833, -13.3628) -> (-19.6833, -5.1171)
  spline S34 degree 2 poles (-19.6833, -5.1171) (-19.4785, -4.8236) (-18.9188, -4.5096) (-18.5707, -4.4618) knots 0 0 0 1 2 2 2
  line L119 (-18.5707, -4.4618) -> (-21.3011, -4.4618)
  line L120 (-21.3011, -4.4618) -> (-21.3011, -10.6461)
  spline S35 degree 2 poles (-21.3011, -10.6461) (-21.9086, -9.4311) (-23.3011, -7.1444) (-24.8642, -5.2468) (-26.6185, -4.025) (-27.5809, -3.8748) knots 0 0 0 1 2 3 4 4 4
  line L121 (-34.4956, -4.4482) -> (-36.3045, -4.4618)
  spline S36 degree 2 poles (-36.3045, -4.4618) (-36.0041, -4.6734) (-35.6697, -5.2741) (-35.6151, -5.6086) knots 0 0 0 1 2 2 2
  spline S37 degree 2 poles (-35.6151, -5.6086) (-35.6151, -6.5369) (-35.6492, -8.3867) (-35.656, -9.3151) knots 0 0 0 1 2 2 2
  line L122 (-35.656, -9.3151) -> (-32.8096, -9.3151)
  spline S38 degree 2 poles (-32.8096, -9.3151) (-33.1577, -9.3082) (-33.4239, -9.0079) (-33.4581, -8.6871) (-33.4649, -8.6529) knots 0 0 0 1 2 3 3 3
  line L123 (-33.4649, -8.6529) -> (-33.4785, -6.5642)
  spline S39 degree 2 poles (-33.4785, -6.5642) (-33.3352, -6.5506) (-33.0826, -6.5369) (-32.9529, -6.5369) knots 0 0 0 1 2 2 2
  spline S40 degree 2 poles (-32.9529, -6.5369) (-31.8813, -6.5506) (-30.4478, -7.3424) (-29.7311, -8.612) (-29.7311, -9.3424) knots 0 0 0 1 2 3 3 3
  spline S41 degree 2 poles (-29.7311, -9.3424) (-29.7311, -10.0591) (-30.4273, -11.3833) (-31.8198, -12.3185) (-32.8642, -12.4618) knots 0 0 0 1 2 3 3 3
  spline S42 degree 2 poles (-32.8642, -12.4618) (-33.1372, -12.5028) (-33.4103, -12.5028) knots 0 0 0 1 1 1
  spline S43 degree 2 poles (-33.4103, -12.5028) (-33.9291, -12.5028) (-35.0417, -12.257) (-35.6014, -11.9908) knots 0 0 0 1 2 2 2
  line L124 (-35.6014, -11.9908) -> (-35.2533, -13.5335)
  spline S44 degree 2 poles (-35.2533, -13.5335) (-35.1099, -13.6359) (-34.3523, -13.8611) (-33.2806, -14.025) (-32.6526, -14.0318) knots 0 0 0 1 2 3 3 3
  spline S45 degree 2 poles (-32.6526, -14.0318) (-31.8198, -14.0386) (-30.0929, -13.6154) (-28.6185, -12.5437) (-27.7106, -10.6393) (-27.6901, -9.1581) knots 0 0 0 1 2 3 4 4 4
  spline S46 degree 2 poles (-27.6901, -9.1581) (-27.7038, -8.3116) (-28.1816, -6.8714) (-28.9325, -5.7997) (-29.3488, -5.5062) knots 0 0 0 1 2 3 3 3
  spline S47 degree 2 poles (-29.3488, -5.5062) (-30.0383, -5.042) (-31.7243, -4.5847) (-33.5741, -4.4413) (-34.4956, -4.4482) knots 0 0 0 1 2 3 3 3
  line L125 (-43.7311, -4.4618) -> (-44.5161, -7.0352)
  spline S48 degree 2 poles (-44.5161, -7.0352) (-44.3796, -6.8236) (-43.3557, -6.5983) (-41.9564, -6.5232) (-41.2396, -6.5232) knots 0 0 0 1 2 3 3 3
  spline S49 degree 2 poles (-41.2396, -6.5232) (-40.5912, -6.5232) (-39.5673, -6.5506) (-39.3079, -6.5506) knots 0 0 0 1 2 2 2
  line L126 (-39.3079, -6.5506) -> (-39.3079, -9.4243)
  line L127 (-39.3079, -9.4243) -> (-41.7516, -9.4243)
  spline S50 degree 2 poles (-41.7516, -9.4243) (-42.086, -9.3355) (-42.5297, -9.0011) (-42.5707, -8.728) knots 0 0 0 1 2 2 2
  line L128 (-42.5707, -8.728) -> (-42.5707, -11.513)
  spline S51 degree 2 poles (-42.5707, -11.513) (-42.5229, -11.24) (-42.1202, -10.8987) (-41.7994, -10.8168) knots 0 0 0 1 2 2 2
  line L129 (-41.7994, -10.8168) -> (-39.3079, -10.8168)
  line L130 (-39.3079, -10.8168) -> (-39.3079, -12.8782)
  spline S52 degree 2 poles (-39.3079, -12.8782) (-39.5195, -12.885) (-40.2499, -12.9123) (-41.1782, -12.9465) (-41.6697, -12.9465) knots 0 0 0 1 2 3 3 3
  spline S53 degree 2 poles (-41.6697, -12.9465) (-42.2499, -12.9465) (-43.2942, -12.8645) (-44.0314, -12.6529) (-44.1543, -12.4482) knots 0 0 0 1 2 3 3 3
  line L131 (-44.1543, -12.4482) -> (-43.7311, -14.0181)
  line L132 (-43.7311, -14.0181) -> (-36.0041, -14.0181)
  spline S54 degree 2 poles (-36.0041, -14.0181) (-36.3523, -13.9703) (-36.912, -13.6495) (-37.1168, -13.3492) knots 0 0 0 1 2 2 2
  line L133 (-37.1168, -13.3492) -> (-37.1168, -5.1171)
  spline S55 degree 2 poles (-37.1168, -5.1171) (-36.912, -4.8236) (-36.3523, -4.5096) (-36.0041, -4.4618) knots 0 0 0 1 2 2 2
  line L134 (-36.0041, -4.4618) -> (-43.7311, -4.4618)
  line L135 (-51.9427, -4.4618) -> (-52.7413, -7.0488)
  spline S56 degree 2 poles (-52.7413, -7.0488) (-52.6048, -6.8304) (-51.6082, -6.6052) (-50.2362, -6.5232) (-49.5331, -6.5232) knots 0 0 0 1 2 3 3 3
  spline S57 degree 2 poles (-49.5331, -6.5232) (-48.8642, -6.5301) (-47.7857, -6.5642) (-47.5195, -6.5642) knots 0 0 0 1 2 2 2
  line L136 (-47.5195, -6.5642) -> (-47.5195, -13.3355)
  spline S58 degree 2 poles (-47.5195, -13.3355) (-47.7311, -13.6427) (-48.2977, -13.9703) (-48.6458, -14.0181) knots 0 0 0 1 2 2 2
  line L137 (-48.6458, -14.0181) -> (-44.2157, -14.0181)
  spline S59 degree 2 poles (-44.2157, -14.0181) (-44.5639, -13.9703) (-45.1304, -13.6427) (-45.342, -13.3355) knots 0 0 0 1 2 2 2
  line L138 (-45.342, -13.3355) -> (-45.342, -5.1512)
  spline S60 degree 2 poles (-45.342, -5.1512) (-45.1304, -4.8441) (-44.5639, -4.5164) (-44.2157, -4.4618) knots 0 0 0 1 2 2 2
  line L139 (-44.2157, -4.4618) -> (-51.9427, -4.4618)
  spline S61 degree 2 poles (-56.871, -4.4618) (-56.5229, -4.5096) (-55.9564, -4.8372) (-55.7448, -5.1444) knots 0 0 0 1 2 2 2
  line L140 (-55.7448, -5.1444) -> (-55.7448, -13.3355)
  spline S62 degree 2 poles (-55.7448, -13.3355) (-55.9564, -13.6427) (-56.5229, -13.9703) (-56.871, -14.0181) knots 0 0 0 1 2 2 2
  line L141 (-56.871, -14.0181) -> (-52.441, -14.0181)
  spline S63 degree 2 poles (-52.441, -14.0181) (-52.7891, -13.9703) (-53.3557, -13.6427) (-53.5673, -13.3355) knots 0 0 0 1 2 2 2
  line L142 (-53.5673, -13.3355) -> (-53.5673, -5.1444)
  spline S64 degree 2 poles (-53.5673, -5.1444) (-53.3557, -4.8372) (-52.7891, -4.5096) (-52.441, -4.4618) knots 0 0 0 1 2 2 2
  line L143 (-52.441, -4.4618) -> (-56.871, -4.4618)
  spline S65 degree 2 poles (-60.8847, -4.4618) (-62.0587, -4.4686) (-63.7584, -5.2331) (-64.8506, -6.5028) (-65.3762, -8.0591) (-65.3762, -8.8645) knots 0 0 0 1 2 3 4 4 4
  spline S66 degree 2 poles (-65.3762, -8.8645) (-65.3762, -9.7929) (-64.7209, -11.4038) (-63.4922, -12.3936) (-62.6253, -12.414) knots 0 0 0 1 2 3 3 3
  spline S67 degree 2 poles (-62.6253, -12.414) (-62.4547, -12.414) (-62.0929, -12.3663) (-61.9017, -12.3185) knots 0 0 0 1 2 2 2
  spline S68 degree 2 poles (-61.9017, -12.3185) (-61.9154, -12.3185) (-62.2977, -11.9157) (-62.7959, -11.1717) (-63.1714, -10.1546) (-63.185, -9.5403) knots 0 0 0 1 2 3 4 4 4
  spline S69 degree 2 poles (-63.185, -9.5403) (-63.185, -9.3424) (-63.1372, -8.9465) (-63.0826, -8.728) knots 0 0 0 1 2 2 2
  spline S70 degree 2 poles (-63.0826, -8.728) (-62.8028, -7.7519) (-61.6697, -6.8236) (-61.0076, -6.8236) knots 0 0 0 1 2 2 2
  spline S71 degree 2 poles (-61.0076, -6.8236) (-60.4478, -6.8304) (-59.4649, -7.4516) (-58.8506, -8.6325) (-58.8369, -9.4721) knots 0 0 0 1 2 3 3 3
  spline S72 degree 2 poles (-58.8369, -9.4721) (-58.8369, -9.8884) (-59.0212, -10.8236) (-59.2192, -11.3424) knots 0 0 0 1 2 2 2
  spline S73 degree 2 poles (-59.2192, -11.3424) (-59.5195, -12.0864) (-60.5502, -12.9396) (-61.6697, -13.3287) (-62.5297, -13.4243) (-62.6594, -13.4174) knots 0 0 0 1 2 3 4 4 4
  line L144 (-62.6594, -13.4174) -> (-62.7004, -13.4174)
  spline S74 degree 2 poles (-62.7004, -13.4174) (-62.4273, -13.786) (-61.5673, -14.025) (-61.069, -14.0181) knots 0 0 0 1 2 2 2
  spline S75 degree 2 poles (-61.069, -14.0181) (-59.9564, -14.0045) (-58.2772, -13.1717) (-57.1372, -11.7587) (-56.5639, -10.0113) (-56.5639, -9.083) knots 0 0 0 1 2 3 4 4 4
  spline S76 degree 2 poles (-56.5639, -9.083) (-56.5639, -8.1956) (-57.0963, -6.5506) (-58.1748, -5.24) (-59.7925, -4.4686) (-60.8847, -4.4618) knots 0 0 0 1 2 3 4 4 4
  spline S77 degree 2 poles (-74.086, -3.8748) (-74.0724, -3.8816) (-73.7311, -4.1683) (-73.3898, -4.6052) (-73.383, -4.8441) knots 0 0 0 1 2 3 3 3
  line L145 (-73.383, -4.8441) -> (-73.383, -13.3355)
  spline S78 degree 2 poles (-73.383, -13.3355) (-73.5878, -13.6427) (-74.1611, -13.9703) (-74.5024, -14.0181) knots 0 0 0 1 2 2 2
  line L146 (-74.5024, -14.0181) -> (-70.6253, -14.0181)
  spline S79 degree 2 poles (-70.6253, -14.0181) (-70.9734, -13.9703) (-71.54, -13.6427) (-71.7516, -13.3355) knots 0 0 0 1 2 2 2
  line L147 (-71.7516, -13.3355) -> (-71.7516, -7.6086)
  spline S80 degree 2 poles (-71.7516, -7.6086) (-71.4171, -8.0727) (-70.5366, -9.6222) (-69.4785, -11.3901) (-68.2703, -12.9874) (-66.9598, -13.9977) (-66.2635, -14.0181) knots 0 0 0 1 2 3 4 5 5 5
  line L148 (-66.2635, -14.0181) -> (-65.0758, -14.0181)
  spline S81 degree 2 poles (-65.0758, -14.0181) (-65.4239, -13.9703) (-65.9837, -13.6564) (-66.1884, -13.3628) knots 0 0 0 1 2 2 2
  line L149 (-66.1884, -13.3628) -> (-66.1884, -5.1171)
  spline S82 degree 2 poles (-66.1884, -5.1171) (-65.9837, -4.8236) (-65.4239, -4.5096) (-65.0758, -4.4618) knots 0 0 0 1 2 2 2
  line L150 (-65.0758, -4.4618) -> (-67.8062, -4.4618)
  line L151 (-67.8062, -4.4618) -> (-67.8062, -10.6461)
  spline S83 degree 2 poles (-67.8062, -10.6461) (-68.4137, -9.4311) (-69.8062, -7.1444) (-71.3693, -5.2468) (-73.1236, -4.025) (-74.086, -3.8748) knots 0 0 0 1 2 3 4 4 4
  point P0 (0, 0)
  point P1 (11.6625, -11.3405)
  point P2 (11.6625, 6.7825)
  point P3 (-78.3875, -11.3405)
  point P4 (-78.3875, 2.7419)
  point P5 (11.6625, -8.9942)
  dimension "d129" = 15
  dimension "d130" = 15
  dimension "d131" = 15
  dimension "d132" = 15
  constraints: 4 point on line, 1 midpoint, 4 other
  measures "d129" distance between parallel lines of L3 L5
  measures "d130" distance between parallel lines of L1 L11
  measures "d131" distance between parallel lines of L10 L5
  measures "d132" distance between parallel lines of L11 L8
extrude "Extrusion4" cut sketch "Sketch4" against normal blind 1.5 contours L16 L17 L18 L19 L20 L21 L22 L23 L24 L25 L26 L27 | L33 L34 L35 L36 L37 L38 L39 L40 | L45 L46 L47 L48 L49 L50 L51 | L62 L63 L64 L65 L66 L67 L68 L69 | L74 L75 L76 L77 | L78 L79 L80 L81 L82 L83 | L84 L85 L86 L87 L88 L89 L90 L91 | L105 S7 L104 S6 L103 L102 S5 S4 L101 L100 S3 L99 S2 L98 L97 S1 S0 L96 | L109 S17 S16 S15 S14 L108 L107 S13 S12 L106 S11 S10 S9 S8 | L112 S34 S18 | S18 S34 L118 S33 L117 S32 L116 S31 L115 S30 L114 S29 S35 L120 L119 | S34 L112 S26 S25 L111 S24 S23 L110 S22 S21 S20 S19 S18 | S47 S46 S45 S44 L124 S43 S42 S41 S40 S39 L123 S38 L122 S37 S36 S55 L134 L121 | L134 S55 S36 | S36 S55 L133 S54 L132 L131 S53 S52 L130 L129 S51 L128 S50 L127 L126 S49 S48 L125 L134 | L139 S60 L138 S59 L137 S58 L136 S57 S56 L135 | L143 S64 L142 S63 L141 S62 L140 S61 | S76 S75 S74 L144 S73 S72 S71 S70 S69 S68 S67 S66 S65 | S83 L151 L150 S82 L149 S81 L148 S80 L147 S79 L146 S78 L145 S77
sketch "Sketch9" plane through (0, 0, 5) normal (0, 0, 1) x (1, 0, 0)
  line L0 (-4.7717, -50.0477) -> (-4.7717, -71.3206) construction
  line L1 (-4.7717, -71.3206) -> (-10.698, -71.3206) construction
  line L2 (-10.698, -71.3206) -> (-10.698, -50.0477) construction
  line L3 (-10.698, -50.0477) -> (-4.7717, -50.0477) construction
  line L4 (-16.1807, -54.1221) -> (-13.2531, -51.6655)
  line L5 (-13.2531, -51.6655) -> (-13.2531, -53.3655)
  line L6 (-13.2531, -53.3655) -> (-11.1807, -53.3655)
  line L7 (-11.1807, -53.3655) -> (-11.1807, -54.8787)
  line L8 (-11.1807, -54.8787) -> (-13.2531, -54.8787)
  line L9 (-13.2531, -54.8787) -> (-13.2531, -56.5787)
  line L10 (-13.2531, -56.5787) -> (-16.1807, -54.1221)
  spline S0 degree 2 poles (-10.4678, -52.3163) (-10.4678, -51.6834) (-10.2227, -50.7296) (-10.0444, -50.3196) knots 0 0 0 1 2 2 2
  line L11 (-10.0444, -50.3196) -> (-8.734, -50.3196)
  line L12 (-8.734, -50.3196) -> (-8.734, -50.4444)
  spline S1 degree 2 poles (-8.734, -50.4444) (-9.0861, -50.8589) (-9.465, -51.8528) (-9.465, -52.3208) knots 0 0 0 1 2 2 2
  spline S2 degree 2 poles (-9.465, -52.3208) (-9.465, -52.4411) (-9.4115, -52.8289) (-9.358, -52.9448) knots 0 0 0 1 2 2 2
  spline S3 degree 2 poles (-9.358, -52.9448) (-9.2956, -53.0874) (-9.0683, -53.288) (-8.8856, -53.288) knots 0 0 0 1 2 2 2
  spline S4 degree 2 poles (-8.8856, -53.288) (-8.6761, -53.288) (-8.4176, -52.9626) (-8.3596, -52.7397) knots 0 0 0 1 2 2 2
  spline S5 degree 2 poles (-8.3596, -52.7397) (-8.2839, -52.4589) (-8.1546, -51.8216) (-8.0566, -51.5408) knots 0 0 0 1 2 2 2
  spline S6 degree 2 poles (-8.0566, -51.5408) (-7.8337, -50.9034) (-7.0716, -50.3508) (-6.5011, -50.3508) knots 0 0 0 1 2 2 2
  spline S7 degree 2 poles (-6.5011, -50.3508) (-5.73, -50.3508) (-4.7717, -51.6567) (-4.7717, -52.6372) knots 0 0 0 1 2 2 2
  spline S8 degree 2 poles (-4.7717, -52.6372) (-4.7717, -53.1275) (-4.9723, -54.0991) (-5.1417, -54.4824) knots 0 0 0 1 2 2 2
  line L13 (-5.1417, -54.4824) -> (-6.3985, -54.4824)
  line L14 (-6.3985, -54.4824) -> (-6.3985, -54.3621)
  spline S9 degree 2 poles (-6.3985, -54.3621) (-6.1356, -54.0546) (-5.7746, -53.1721) (-5.7746, -52.7085) knots 0 0 0 1 2 2 2
  spline S10 degree 2 poles (-5.7746, -52.7085) (-5.7746, -52.5258) (-5.828, -52.2405) (-5.8994, -52.0801) knots 0 0 0 1 2 2 2
  spline S11 degree 2 poles (-5.8994, -52.0801) (-5.9573, -51.9508) (-6.1891, -51.7636) (-6.3317, -51.7636) knots 0 0 0 1 2 2 2
  spline S12 degree 2 poles (-6.3317, -51.7636) (-6.5456, -51.7636) (-6.7908, -52.0623) (-6.8888, -52.4901) knots 0 0 0 1 2 2 2
  spline S13 degree 2 poles (-6.8888, -52.4901) (-6.9512, -52.7665) (-7.0716, -53.279) (-7.1741, -53.5732) knots 0 0 0 1 2 2 2
  spline S14 degree 2 poles (-7.1741, -53.5732) (-7.3836, -54.1437) (-8.0789, -54.7008) (-8.6494, -54.7008) knots 0 0 0 1 2 2 2
  spline S15 degree 2 poles (-8.6494, -54.7008) (-9.4695, -54.7008) (-10.4678, -53.4128) (-10.4678, -52.3163) knots 0 0 0 1 2 2 2
  line L15 (-10.3698, -56.4658) -> (-5.9172, -56.4658)
  line L16 (-5.9172, -56.4658) -> (-5.9172, -54.839)
  line L17 (-5.9172, -54.839) -> (-4.8698, -54.839)
  line L18 (-4.8698, -54.839) -> (-4.8698, -59.4743)
  line L19 (-4.8698, -59.4743) -> (-5.9172, -59.4743)
  line L20 (-5.9172, -59.4743) -> (-5.9172, -57.8475)
  line L21 (-5.9172, -57.8475) -> (-10.3698, -57.8475)
  line L22 (-10.3698, -57.8475) -> (-10.3698, -56.4658)
  line L23 (-10.3698, -59.4476) -> (-4.8698, -61.3062)
  line L24 (-4.8698, -61.3062) -> (-4.8698, -62.8127)
  line L25 (-4.8698, -62.8127) -> (-10.3698, -64.6713)
  line L26 (-10.3698, -64.6713) -> (-10.3698, -63.2495)
  line L27 (-10.3698, -63.2495) -> (-9.2466, -62.9063)
  line L28 (-9.2466, -62.9063) -> (-9.2466, -61.1769)
  line L29 (-9.2466, -61.1769) -> (-10.3698, -60.8293)
  line L30 (-10.3698, -60.8293) -> (-10.3698, -59.4476)
  line L31 (-8.2482, -62.6032) -> (-6.4297, -62.0416)
  line L32 (-6.4297, -62.0416) -> (-8.2482, -61.4756)
  line L33 (-8.2482, -61.4756) -> (-8.2482, -62.6032)
  line L34 (-10.3698, -70.3005) -> (-10.3698, -68.6202)
  line L35 (-10.3698, -68.6202) -> (-8.3507, -67.0914)
  line L36 (-8.3507, -67.0914) -> (-8.3507, -66.5922)
  line L37 (-8.3507, -66.5922) -> (-10.3698, -66.5922)
  line L38 (-10.3698, -66.5922) -> (-10.3698, -65.2195)
  line L39 (-10.3698, -65.2195) -> (-4.8698, -65.2195)
  line L40 (-4.8698, -65.2195) -> (-4.8698, -67.4302)
  spline S16 degree 2 poles (-4.8698, -67.4302) (-4.8698, -67.8893) (-4.9857, -68.5667) (-5.1639, -68.8564) knots 0 0 0 1 2 2 2
  spline S17 degree 2 poles (-5.1639, -68.8564) (-5.3511, -69.1506) (-5.935, -69.4982) (-6.3807, -69.4982) knots 0 0 0 1 2 2 2
  spline S18 degree 2 poles (-6.3807, -69.4982) (-7.0092, -69.4982) (-7.7981, -68.9277) (-8.0298, -68.4508) knots 0 0 0 1 2 2 2
  line L41 (-8.0298, -68.4508) -> (-10.3698, -70.3005)
  spline S19 degree 2 poles (-6.5545, -68.0809) (-6.3451, -68.0809) (-6.0464, -67.9205) (-5.9662, -67.7377) knots 0 0 0 1 2 2 2
  spline S20 degree 2 poles (-5.9662, -67.7377) (-5.9127, -67.6085) (-5.8815, -67.292) (-5.8815, -67.0558) knots 0 0 0 1 2 2 2
  line L42 (-5.8815, -67.0558) -> (-5.8815, -66.5922)
  line L43 (-5.8815, -66.5922) -> (-7.3613, -66.5922)
  line L44 (-7.3613, -66.5922) -> (-7.3613, -66.9889)
  spline S21 degree 2 poles (-7.3613, -66.9889) (-7.3613, -67.2742) (-7.29, -67.6798) (-7.1785, -67.8179) knots 0 0 0 1 2 2 2
  spline S22 degree 2 poles (-7.1785, -67.8179) (-7.0716, -67.9517) (-6.7863, -68.0809) (-6.5545, -68.0809) knots 0 0 0 1 2 2 2
  line L45 (-10.3698, -71.7669) -> (-5.9172, -71.7669)
  line L46 (-5.9172, -71.7669) -> (-5.9172, -70.1401)
  line L47 (-5.9172, -70.1401) -> (-4.8698, -70.1401)
  line L48 (-4.8698, -70.1401) -> (-4.8698, -74.7754)
  line L49 (-4.8698, -74.7754) -> (-5.9172, -74.7754)
  line L50 (-5.9172, -74.7754) -> (-5.9172, -73.1486)
  line L51 (-5.9172, -73.1486) -> (-10.3698, -73.1486)
  line L52 (-10.3698, -73.1486) -> (-10.3698, -71.7669)
  point P0 (0, 0)
  dimension "d121" = 50
  dimension "d122" = 50
  dimension "d124" = 1.7
  dimension "d125" = 1.7
  dimension "d126" = 5
  constraints: 14 end point, 3 vertical, 2 horizontal, 1 parallel, 1 point on line, 3 other
  measures "d121" angle of L5 L4
  measures "d122" angle of L9 L10
  measures "d124" distance of L4.end L5.end
  measures "d125" distance of L8.end L9.end
  measures "d126" distance from line of L4.start L7
extrude "Extrusion8" cut sketch "Sketch9" against normal blind 1.5
body "Solid1"
